Autodesk Fusion 360 part; units mm, degrees
(part 23 of 24)
  arc A327 (62.8291, 5.0441) -> (62.9009, 5.1159) centre (62.865, 5.08) ccw
  arc A328 (66.675, 5.0292) -> (66.675, 5.1308) centre (66.675, 5.08) ccw
  line L165 (33.655, 7.62) -> (32.385, 7.62)
  line L166 (34.29, 5.715) -> (34.925, 5.08)
  line L167 (36.195, 7.62) -> (34.925, 7.62)
  line L168 (64.135, 7.62) -> (62.865, 7.62)
  arc A329 (62.865, 7.6708) -> (62.865, 7.5692) centre (62.865, 7.62) ccw
  arc A330 (31.6992, 5.715) -> (31.8008, 5.715) centre (31.75, 5.715) ccw
  line L169 (56.515, 7.62) -> (55.245, 7.62)
  line L170 (57.785, 5.08) -> (59.055, 5.08)
  arc A331 (57.7491, 5.0441) -> (57.8209, 5.1159) centre (57.785, 5.08) ccw
  arc A332 (64.135, 7.5692) -> (64.135, 7.6708) centre (64.135, 7.62) ccw
  arc A333 (62.2659, 5.6791) -> (62.1941, 5.7509) centre (62.23, 5.715) ccw
  arc A334 (65.405, 7.6708) -> (65.405, 7.5692) centre (65.405, 7.62) ccw
  arc A335 (59.0909, 7.6559) -> (59.0191, 7.5841) centre (59.055, 7.62) ccw
  arc A336 (54.5741, 7.0209) -> (54.6459, 6.9491) centre (54.61, 6.985) ccw
  arc A337 (61.595, 7.5692) -> (61.595, 7.6708) centre (61.595, 7.62) ccw
  line L171 (60.325, 7.62) -> (59.69, 6.985)
  arc A338 (64.8059, 5.7509) -> (64.7341, 5.6791) centre (64.77, 5.715) ccw
  arc A339 (56.4791, 5.1159) -> (56.5509, 5.0441) centre (56.515, 5.08) ccw
  arc A340 (66.675, 7.5692) -> (66.675, 7.6708) centre (66.675, 7.62) ccw
  line L172 (62.865, 7.62) -> (62.23, 6.985)
  arc A341 (60.2891, 5.0441) -> (60.3609, 5.1159) centre (60.325, 5.08) ccw
  arc A342 (59.6541, 6.9491) -> (59.7259, 7.0209) centre (59.69, 6.985) ccw
  arc A343 (64.7341, 7.0209) -> (64.8059, 6.9491) centre (64.77, 6.985) ccw
  arc A344 (57.1141, 6.9491) -> (57.1859, 7.0209) centre (57.15, 6.985) ccw
  line L173 (60.325, 5.08) -> (61.595, 5.08)
  line L174 (59.69, 6.985) -> (59.055, 7.62)
  arc A345 (61.5591, 5.1159) -> (61.6309, 5.0441) centre (61.595, 5.08) ccw
  arc A346 (60.325, 5.1308) -> (60.325, 5.0292) centre (60.325, 5.08) ccw
  arc A347 (57.785, 5.1308) -> (57.785, 5.0292) centre (57.785, 5.08) ccw
  arc A348 (62.9009, 7.5841) -> (62.8291, 7.6559) centre (62.865, 7.62) ccw
  line L175 (66.675, 7.62) -> (65.405, 7.62)
  arc A349 (55.245, 7.6708) -> (55.245, 7.5692) centre (55.245, 7.62) ccw
  line L176 (61.595, 7.62) -> (60.325, 7.62)
  arc A350 (56.515, 7.5692) -> (56.515, 7.6708) centre (56.515, 7.62) ccw
  arc A351 (59.6541, 7.0209) -> (59.7259, 6.9491) centre (59.69, 6.985) ccw
  arc A352 (65.3691, 5.0441) -> (65.4409, 5.1159) centre (65.405, 5.08) ccw
  line L177 (61.595, 5.08) -> (62.23, 5.715)
  arc A353 (55.2091, 5.0441) -> (55.2809, 5.1159) centre (55.245, 5.08) ccw
  arc A354 (53.975, 5.0292) -> (53.975, 5.1308) centre (53.975, 5.08) ccw
  arc A355 (57.1141, 7.0209) -> (57.1859, 6.9491) centre (57.15, 6.985) ccw
  line L178 (64.77, 6.985) -> (65.405, 7.62)
  arc A356 (59.7259, 5.6791) -> (59.6541, 5.7509) centre (59.69, 5.715) ccw
  arc A357 (59.7259, 5.7509) -> (59.6541, 5.6791) centre (59.69, 5.715) ccw
  arc A358 (60.325, 7.6708) -> (60.325, 7.5692) centre (60.325, 7.62) ccw
  arc A359 (57.8209, 7.5841) -> (57.7491, 7.6559) centre (57.785, 7.62) ccw
  arc A360 (69.8141, 6.9491) -> (69.8859, 7.0209) centre (69.85, 6.985) ccw
  line L179 (62.23, 6.985) -> (61.595, 7.62)
  arc A361 (62.1941, 6.9491) -> (62.2659, 7.0209) centre (62.23, 6.985) ccw
  arc A362 (62.1941, 7.0209) -> (62.2659, 6.9491) centre (62.23, 6.985) ccw
  line L180 (57.15, 6.985) -> (57.785, 7.62)
  line L181 (57.785, 5.08) -> (57.15, 5.715)
  line L182 (55.245, 7.62) -> (54.61, 6.985)
  arc A363 (60.3609, 7.5841) -> (60.2891, 7.6559) centre (60.325, 7.62) ccw
  arc A364 (61.6309, 7.6559) -> (61.5591, 7.5841) centre (61.595, 7.62) ccw
  arc A365 (56.515, 5.0292) -> (56.515, 5.1308) centre (56.515, 5.08) ccw
  arc A366 (57.1859, 5.7509) -> (57.1141, 5.6791) centre (57.15, 5.715) ccw
  arc A367 (55.2809, 7.5841) -> (55.2091, 7.6559) centre (55.245, 7.62) ccw
  line L183 (65.405, 5.08) -> (64.77, 5.715)
sketch "Bottom Silkscreen" plane through (0, 0, 0) normal (0, 0, 1) x (1, 0, 0)
  arc A0 (64.6974, 49.0665) -> (64.6974, 49.1553) centre (64.6974, 49.1109) ccw
  arc A1 (63.764, 50.3111) -> (63.8529, 50.3111) centre (63.8085, 50.3111) ccw
  arc A2 (63.8084, 50.3111) -> (63.9418, 49.9999) centre (64.2381, 50.3111) ccw
  arc A3 (63.9756, 50.0287) -> (63.9079, 49.9711) centre (63.9418, 49.9999) ccw
  arc A4 (63.8529, 50.3111) -> (63.764, 50.311) centre (63.8085, 50.311) ccw
  arc A5 (65.4177, 49.4665) -> (65.7733, 49.1109) centre (65.7733, 49.4665) ccw
  arc A6 (64.6974, 50.3555) -> (64.2085, 50.7111) centre (64.2085, 50.1972) ccw
  arc A7 (65.4621, 49.4665) -> (65.3732, 49.4665) centre (65.4177, 49.4665) ccw
  arc A8 (65.7733, 49.1553) -> (65.7733, 49.0665) centre (65.7733, 49.1109) ccw
  line L0 (63.9418, 49.9999) -> (64.6974, 49.1109)
  arc A9 (64.2085, 50.7555) -> (64.2085, 50.6667) centre (64.2085, 50.7111) ccw
  arc A10 (64.6551, 50.3418) -> (64.7397, 50.3692) centre (64.6974, 50.3555) ccw
  arc A11 (64.6636, 49.0821) -> (64.7313, 49.1397) centre (64.6975, 49.1109) ccw
  line L1 (65.7733, 49.1109) -> (65.9511, 49.1109)
  arc A12 (63.8084, 49.1553) -> (63.8084, 49.0665) centre (63.8084, 49.1109) ccw
  arc A13 (65.9511, 49.0665) -> (65.9511, 49.1553) centre (65.9511, 49.1109) ccw
  arc A14 (63.9111, 49.9677) -> (63.9724, 50.0321) centre (63.9418, 49.9999) ccw
  arc A15 (64.2085, 50.7111) -> (63.8084, 50.3111) centre (64.2085, 50.311) ccw
  line L2 (64.6974, 49.1109) -> (63.8084, 49.1109)
  arc A16 (65.4621, 50.7111) -> (65.3732, 50.7111) centre (65.4177, 50.7111) ccw
  arc A17 (28.0289, 5.2134) -> (28.0289, 5.1244) centre (28.0289, 5.1689) ccw
  arc A18 (29.9938, 5.2134) -> (29.9938, 5.1244) centre (29.9938, 5.1689) ccw
  arc A19 (28.9179, 5.1244) -> (28.9179, 5.2134) centre (28.9179, 5.1689) ccw
  line L3 (29.9938, 5.1689) -> (30.1716, 5.1689)
  arc A20 (28.5179, 6.7691) -> (28.429, 6.7691) centre (28.4735, 6.7691) ccw
  arc A21 (29.6382, 5.5245) -> (29.9938, 5.1689) centre (29.9938, 5.5245) ccw
  arc A22 (28.5012, 6.8038) -> (28.4456, 6.7344) centre (28.4734, 6.7691) ccw
  line L4 (28.9179, 5.1689) -> (28.0289, 5.1689)
  line L5 (28.4734, 6.7691) -> (28.4734, 5.1689)
  arc A23 (29.9938, 5.1244) -> (29.9938, 5.2134) centre (29.9938, 5.1689) ccw
  arc A24 (28.429, 5.1689) -> (28.5179, 5.1689) centre (28.4735, 5.1689) ccw
  arc A25 (30.1716, 5.1244) -> (30.1716, 5.2134) centre (30.1716, 5.1689) ccw
  arc A26 (29.5937, 5.5245) -> (29.6826, 5.5245) centre (29.6382, 5.5245) ccw
  arc A27 (29.6826, 5.5245) -> (29.5937, 5.5245) centre (29.6382, 5.5245) ccw
  arc A28 (64.2085, 50.6667) -> (64.2085, 50.7555) centre (64.2085, 50.7111) ccw
  arc A29 (65.3732, 49.4665) -> (65.4621, 49.4665) centre (65.4177, 49.4665) ccw
  arc A30 (28.8901, 6.3788) -> (28.9457, 6.4482) centre (28.9179, 6.4135) ccw
  arc A31 (29.6826, 6.7691) -> (29.5937, 6.7691) centre (29.6382, 6.7691) ccw
  line L6 (65.4177, 50.7111) -> (65.4177, 49.4665)
  arc A32 (65.7733, 49.0665) -> (65.7733, 49.1553) centre (65.7733, 49.1109) ccw
  line L7 (29.6382, 6.7691) -> (29.6382, 5.5245)
  line L8 (28.9179, 6.4135) -> (28.4734, 6.7691)
sketch "Top Traces]" plane through (0, 0, 0) normal (0, 0, 1) x (1, 0, 0)
  arc A0 (58.4962, 25.4) -> (58.3438, 25.4) centre (58.42, 25.4) ccw
  arc A1 (31.6738, 22.86) -> (31.8262, 22.86) centre (31.75, 22.86) ccw
  line L0 (29.21, 10.16) -> (44.45, 10.16)
  arc A2 (26.67, 21.6662) -> (26.67, 21.5138) centre (26.67, 21.59) ccw
  arc A3 (30.48, 21.5138) -> (30.48, 21.6662) centre (30.48, 21.59) ccw
  line L1 (58.42, 16.51) -> (55.88, 13.97)
  arc A4 (29.21, 10.2362) -> (29.21, 10.0838) centre (29.21, 10.16) ccw
  arc A5 (44.5039, 10.2139) -> (44.3961, 10.1061) centre (44.45, 10.16) ccw
  line L2 (46.99, 11.43) -> (48.26, 10.16)
  arc A6 (45.6438, 6.35) -> (45.7962, 6.35) centre (45.72, 6.35) ccw
  arc A7 (58.4962, 20.32) -> (58.3438, 20.32) centre (58.42, 20.32) ccw
  arc A8 (46.99, 11.3538) -> (46.99, 11.5062) centre (46.99, 11.43) ccw
  line L3 (27.94, 16.51) -> (27.94, 19.05)
  arc A9 (25.3238, 13.97) -> (25.4762, 13.97) centre (25.4, 13.97) ccw
  arc A10 (48.3362, 10.16) -> (48.1838, 10.16) centre (48.26, 10.16) ccw
  arc A11 (28.0162, 19.05) -> (27.8638, 19.05) centre (27.94, 19.05) ccw
  line L4 (25.4, 13.97) -> (29.21, 10.16)
  line L5 (30.48, 11.43) -> (46.99, 11.43)
  line L6 (26.67, 21.59) -> (30.48, 21.59)
  arc A12 (25.3461, 20.3739) -> (25.4539, 20.2661) centre (25.4, 20.32) ccw
  line L7 (55.88, 13.97) -> (45.72, 13.97)
  arc A13 (48.2061, 10.1061) -> (48.3139, 10.2139) centre (48.26, 10.16) ccw
  arc A14 (25.3238, 16.51) -> (25.4762, 16.51) centre (25.4, 16.51) ccw
  arc A15 (58.3438, 16.51) -> (58.4962, 16.51) centre (58.42, 16.51) ccw
  line L8 (58.42, 20.32) -> (58.42, 16.51)
  arc A16 (26.7239, 21.5361) -> (26.6161, 21.6439) centre (26.67, 21.59) ccw
  line L9 (27.94, 13.97) -> (30.48, 11.43)
  arc A17 (44.45, 10.0838) -> (44.45, 10.2362) centre (44.45, 10.16) ccw
  arc A18 (45.7962, 8.89) -> (45.6438, 8.89) centre (45.72, 8.89) ccw
  arc A19 (30.4261, 21.6439) -> (30.5339, 21.5361) centre (30.48, 21.59) ccw
  arc A20 (25.4539, 14.0239) -> (25.3461, 13.9161) centre (25.4, 13.97) ccw
  line L10 (27.94, 16.51) -> (27.94, 13.97)
  arc A21 (29.1561, 10.1061) -> (29.2639, 10.2139) centre (29.21, 10.16) ccw
  arc A22 (31.8039, 22.8061) -> (31.6961, 22.9139) centre (31.75, 22.86) ccw
  line L11 (44.45, 10.16) -> (45.72, 8.89)
  arc A23 (63.6587, 35.56) -> (63.3413, 35.56) centre (63.5, 35.56) ccw
  line L12 (25.4, 16.51) -> (25.4, 13.97)
  arc A24 (55.88, 13.8938) -> (55.88, 14.0462) centre (55.88, 13.97) ccw
  line L13 (25.4, 16.51) -> (25.4, 20.32)
  line L14 (30.48, 21.59) -> (31.75, 22.86)
  arc A25 (27.9939, 14.0239) -> (27.8861, 13.9161) centre (27.94, 13.97) ccw
  arc A26 (30.4261, 11.3761) -> (30.5339, 11.4839) centre (30.48, 11.43) ccw
  arc A27 (45.72, 14.0462) -> (45.72, 13.8938) centre (45.72, 13.97) ccw
  line L15 (45.72, 8.89) -> (45.72, 6.35)
  line L16 (31.75, 22.86) -> (31.75, 25.4)
  arc A28 (25.4762, 16.51) -> (25.3238, 16.51) centre (25.4, 16.51) ccw
  line L17 (25.4, 20.32) -> (26.67, 21.59)
  arc A29 (27.8638, 16.51) -> (28.0162, 16.51) centre (27.94, 16.51) ccw
  arc A30 (47.0439, 11.4839) -> (46.9361, 11.3761) centre (46.99, 11.43) ccw
  arc A31 (58.4739, 16.4561) -> (58.3661, 16.5639) centre (58.42, 16.51) ccw
  arc A32 (15.8897, 25.7957) -> (16.1143, 26.0203) centre (16.002, 25.908) ccw
  arc A33 (30.48, 11.5062) -> (30.48, 11.3538) centre (30.48, 11.43) ccw
  arc A34 (40.7987, 38.1) -> (40.4813, 38.1) centre (40.64, 38.1) ccw
  arc A35 (48.1838, 6.35) -> (48.3362, 6.35) centre (48.26, 6.35) ccw
  arc A36 (15.3523, 26.7823) -> (15.1277, 26.5577) centre (15.24, 26.67) ccw
  arc A37 (45.6661, 8.8361) -> (45.7739, 8.9439) centre (45.72, 8.89) ccw
  arc A38 (28.0162, 16.51) -> (27.8638, 16.51) centre (27.94, 16.51) ccw
  line L18 (58.42, 25.4) -> (58.42, 20.32)
  line L19 (48.26, 10.16) -> (48.26, 6.35)
  arc A39 (30.5562, 17.78) -> (30.4038, 17.78) centre (30.48, 17.78) ccw
  line L20 (49.53, 12.7) -> (50.8, 11.43)
  arc A40 (31.8231, 20.3739) -> (31.9309, 20.2661) centre (31.877, 20.32) ccw
  line L21 (31.75, 12.7) -> (49.53, 12.7)
  line L22 (76.2, 29.718) -> (75.692, 29.21)
  arc A41 (70.0309, 29.1561) -> (69.9231, 29.2639) centre (69.977, 29.21) ccw
  arc A42 (36.9062, 25.4) -> (36.7538, 25.4) centre (36.83, 25.4) ccw
  line L23 (30.48, 16.51) -> (30.48, 13.97)
  arc A43 (33.02, 18.9738) -> (33.02, 19.1262) centre (33.02, 19.05) ccw
  arc A44 (55.8261, 14.0239) -> (55.9339, 13.9161) centre (55.88, 13.97) ccw
  arc A45 (36.8839, 22.8061) -> (36.7761, 22.9139) centre (36.83, 22.86) ccw
  line L24 (31.75, 19.05) -> (33.02, 19.05)
  line L25 (60.96, 25.4) -> (60.96, 15.24)
  arc A46 (30.5562, 16.51) -> (30.4038, 16.51) centre (30.48, 16.51) ccw
  arc A47 (25.4762, 20.32) -> (25.3238, 20.32) centre (25.4, 20.32) ccw
  arc A48 (61.0362, 25.4) -> (60.8838, 25.4) centre (60.96, 25.4) ccw
  arc A49 (30.4261, 17.8339) -> (30.5339, 17.7261) centre (30.48, 17.78) ccw
  line L26 (33.02, 19.05) -> (36.83, 22.86)
  arc A50 (50.8762, 11.43) -> (50.7238, 11.43) centre (50.8, 11.43) ccw
  line L27 (34.29, 22.733) -> (34.29, 25.4)
  arc A51 (50.7238, 6.35) -> (50.8762, 6.35) centre (50.8, 6.35) ccw
  line L28 (76.2, 31.75) -> (76.2, 29.718)
  arc A52 (34.3439, 22.6791) -> (34.2361, 22.7869) centre (34.29, 22.733) ccw
  arc A53 (27.8861, 19.1039) -> (27.9939, 18.9961) centre (27.94, 19.05) ccw
  line L29 (75.692, 29.21) -> (69.977, 29.21)
  arc A54 (58.3438, 20.32) -> (58.4962, 20.32) centre (58.42, 20.32) ccw
  arc A55 (31.8262, 25.4) -> (31.6738, 25.4) centre (31.75, 25.4) ccw
  arc A56 (75.6381, 29.2639) -> (75.7459, 29.1561) centre (75.692, 29.21) ccw
  arc A57 (76.2762, 31.75) -> (76.1238, 31.75) centre (76.2, 31.75) ccw
  line L30 (31.877, 20.32) -> (34.29, 22.733)
  line L31 (30.48, 13.97) -> (31.75, 12.7)
  arc A58 (58.3661, 12.7539) -> (58.4739, 12.6461) centre (58.42, 12.7) ccw
  arc A59 (61.0139, 15.1861) -> (60.9061, 15.2939) centre (60.96, 15.24) ccw
  arc A60 (69.2881, 28.6289) -> (69.3959, 28.5211) centre (69.342, 28.575) ccw
  arc A61 (30.4038, 13.97) -> (30.5562, 13.97) centre (30.48, 13.97) ccw
  arc A62 (27.8638, 13.97) -> (28.0162, 13.97) centre (27.94, 13.97) ccw
  arc A63 (29.2639, 20.2661) -> (29.1561, 20.3739) centre (29.21, 20.32) ccw
  line L32 (58.42, 12.7) -> (55.88, 12.7)
  arc A64 (49.53, 12.6238) -> (49.53, 12.7762) centre (49.53, 12.7) ccw
  arc A65 (49.5839, 12.7539) -> (49.4761, 12.6461) centre (49.53, 12.7) ccw
  arc A66 (75.692, 29.1338) -> (75.692, 29.2862) centre (75.692, 29.21) ccw
  arc A67 (69.977, 29.2862) -> (69.977, 29.1338) centre (69.977, 29.21) ccw
  arc A68 (31.75, 19.1262) -> (31.75, 18.9738) centre (31.75, 19.05) ccw
  line L33 (69.977, 29.21) -> (69.342, 28.575)
  line L34 (60.96, 15.24) -> (58.42, 12.7)
  line L35 (30.48, 17.78) -> (31.75, 19.05)
  arc A69 (50.7461, 11.3761) -> (50.8539, 11.4839) centre (50.8, 11.43) ccw
  line L36 (30.48, 16.51) -> (30.48, 17.78)
  line L37 (36.83, 22.86) -> (36.83, 25.4)
  arc A70 (31.877, 20.2438) -> (31.877, 20.3962) centre (31.877, 20.32) ccw
  arc A71 (31.8039, 18.9961) -> (31.6961, 19.1039) centre (31.75, 19.05) ccw
  arc A72 (76.1238, 29.718) -> (76.2762, 29.718) centre (76.2, 29.718) ccw
  arc A73 (34.3662, 25.4) -> (34.2138, 25.4) centre (34.29, 25.4) ccw
  arc A74 (36.7538, 22.86) -> (36.9062, 22.86) centre (36.83, 22.86) ccw
  arc A75 (32.9661, 19.1039) -> (33.0739, 18.9961) centre (33.02, 19.05) ccw
  arc A76 (60.8838, 15.24) -> (61.0362, 15.24) centre (60.96, 15.24) ccw
  arc A77 (34.2138, 22.733) -> (34.3662, 22.733) centre (34.29, 22.733) ccw
  arc A78 (76.2539, 29.6641) -> (76.1461, 29.7719) centre (76.2, 29.718) ccw
  arc A79 (29.21, 20.3962) -> (29.21, 20.2438) centre (29.21, 20.32) ccw
  line L38 (27.94, 19.05) -> (29.21, 20.32)
  arc A80 (62.1761, 24.1839) -> (62.2839, 24.0761) centre (62.23, 24.13) ccw
  line L39 (76.2, 40.64) -> (76.2, 44.45)
  arc A81 (76.2539, 40.5861) -> (76.1461, 40.6939) centre (76.2, 40.64) ccw
  arc A82 (60.9061, 25.4539) -> (61.0139, 25.3461) centre (60.96, 25.4) ccw
  line L40 (55.88, 10.16) -> (57.15, 11.43)
  line L41 (62.23, 13.97) -> (62.23, 24.13)
  arc A83 (62.1538, 13.97) -> (62.3062, 13.97) centre (62.23, 13.97) ccw
  line L42 (50.8, 11.43) -> (50.8, 6.35)
  line L43 (65.405, 27.305) -> (70.485, 27.305)
  line L44 (69.342, 28.575) -> (64.135, 28.575)
  line L45 (57.15, 11.43) -> (59.69, 11.43)
  arc A84 (76.2762, 44.45) -> (76.1238, 44.45) centre (76.2, 44.45) ccw
  arc A85 (77.4161, 27.9939) -> (77.5239, 27.8861) centre (77.47, 27.94) ccw
  arc A86 (58.42, 12.6238) -> (58.42, 12.7762) centre (58.42, 12.7) ccw
  line L46 (53.34, 10.16) -> (53.34, 6.35)
  arc A87 (74.8761, 39.4239) -> (74.9839, 39.3161) centre (74.93, 39.37) ccw
  line L47 (71.12, 39.37) -> (74.93, 39.37)
  line L48 (55.88, 6.35) -> (55.88, 10.16)
  arc A88 (57.15, 11.5062) -> (57.15, 11.3538) centre (57.15, 11.43) ccw
  arc A89 (62.2839, 13.9161) -> (62.1761, 14.0239) centre (62.23, 13.97) ccw
  arc A90 (74.93, 39.2938) -> (74.93, 39.4462) centre (74.93, 39.37) ccw
  arc A91 (55.9562, 10.16) -> (55.8038, 10.16) centre (55.88, 10.16) ccw
  line L49 (29.21, 20.32) -> (31.877, 20.32)
  arc A92 (64.1889, 28.5211) -> (64.0811, 28.6289) centre (64.135, 28.575) ccw
  arc A93 (53.2861, 10.2139) -> (53.3939, 10.1061) centre (53.34, 10.16) ccw
  arc A94 (71.12, 39.4462) -> (71.12, 39.2938) centre (71.12, 39.37) ccw
  arc A95 (76.1238, 40.64) -> (76.2762, 40.64) centre (76.2, 40.64) ccw
  arc A96 (65.4589, 27.2511) -> (65.3511, 27.3589) centre (65.405, 27.305) ccw
  line L50 (62.23, 24.13) -> (65.405, 27.305)
  arc A97 (71.1739, 27.8861) -> (71.0661, 27.9939) centre (71.12, 27.94) ccw
  arc A98 (30.4038, 16.51) -> (30.5562, 16.51) centre (30.48, 16.51) ccw
  line L51 (70.485, 27.305) -> (71.12, 27.94)
  arc A99 (70.485, 27.2288) -> (70.485, 27.3812) centre (70.485, 27.305) ccw
  arc A100 (77.47, 27.8638) -> (77.47, 28.0162) centre (77.47, 27.94) ccw
  line L52 (55.88, 12.7) -> (53.34, 10.16)
  arc A101 (59.69, 11.3538) -> (59.69, 11.5062) centre (59.69, 11.43) ccw
  arc A102 (59.6361, 11.4839) -> (59.7439, 11.3761) centre (59.69, 11.43) ccw
  arc A103 (55.88, 12.7762) -> (55.88, 12.6238) centre (55.88, 12.7) ccw
  arc A104 (64.135, 28.6512) -> (64.135, 28.4988) centre (64.135, 28.575) ccw
  arc A105 (55.8038, 6.35) -> (55.9562, 6.35) centre (55.88, 6.35) ccw
  arc A106 (31.75, 12.7762) -> (31.75, 12.6238) centre (31.75, 12.7) ccw
  arc A107 (69.342, 28.4988) -> (69.342, 28.6512) centre (69.342, 28.575) ccw
  arc A108 (55.8261, 10.2139) -> (55.9339, 10.1061) centre (55.88, 10.16) ccw
  arc A109 (30.5339, 14.0239) -> (30.4261, 13.9161) centre (30.48, 13.97) ccw
  arc A110 (62.3062, 24.13) -> (62.1538, 24.13) centre (62.23, 24.13) ccw
  arc A111 (31.6961, 12.6461) -> (31.8039, 12.7539) centre (31.75, 12.7) ccw
  arc A112 (53.4162, 10.16) -> (53.2638, 10.16) centre (53.34, 10.16) ccw
  arc A113 (55.9339, 12.6461) -> (55.8261, 12.7539) centre (55.88, 12.7) ccw
  arc A114 (65.405, 27.3812) -> (65.405, 27.2288) centre (65.405, 27.305) ccw
  arc A115 (53.2638, 6.35) -> (53.4162, 6.35) centre (53.34, 6.35) ccw
  arc A116 (70.4311, 27.3589) -> (70.5389, 27.2511) centre (70.485, 27.305) ccw
  line L53 (64.135, 28.575) -> (60.96, 25.4)
  line L54 (74.93, 39.37) -> (76.2, 40.64)
  arc A117 (57.2039, 11.3761) -> (57.0961, 11.4839) centre (57.15, 11.43) ccw
  line L55 (59.69, 11.43) -> (62.23, 13.97)
  line L56 (71.12, 27.94) -> (77.47, 27.94)
  line L57 (3.048, 46.228) -> (3.81, 46.99)
  line L58 (3.81, 46.99) -> (8.89, 46.99)
  arc A118 (60.96, 31.6738) -> (60.96, 31.8262) centre (60.96, 31.75) ccw
  arc A119 (55.8038, 34.29) -> (55.9562, 34.29) centre (55.88, 34.29) ccw
  line L59 (60.96, 31.75) -> (54.61, 31.75)
  line L60 (3.048, 44.45) -> (3.048, 46.228)
  arc A120 (16.5862, 49.53) -> (16.4338, 49.53) centre (16.51, 49.53) ccw
  line L61 (76.327, 36.83) -> (78.74, 39.243)
  arc A121 (10.16, 45.7962) -> (10.16, 45.6438) centre (10.16, 45.72) ccw
  line L62 (15.24, 45.72) -> (16.51, 46.99)
  arc A122 (71.12, 36.9062) -> (71.12, 36.7538) centre (71.12, 36.83) ccw
  arc A123 (76.327, 36.7538) -> (76.327, 36.9062) centre (76.327, 36.83) ccw
  arc A124 (78.6638, 39.243) -> (78.8162, 39.243) centre (78.74, 39.243) ccw
  line L63 (71.12, 36.83) -> (76.327, 36.83)
  line L64 (67.31, 16.51) -> (67.31, 10.16)
  arc A125 (78.8162, 44.45) -> (78.6638, 44.45) centre (78.74, 44.45) ccw
  arc A126 (78.6638, 29.21) -> (78.8162, 29.21) centre (78.74, 29.21) ccw
  arc A127 (8.89, 46.9138) -> (8.89, 47.0662) centre (8.89, 46.99) ccw
  arc A128 (3.1242, 46.228) -> (2.9718, 46.228) centre (3.048, 46.228) ccw
  arc A129 (2.9718, 44.45) -> (3.1242, 44.45) centre (3.048, 44.45) ccw
  line L65 (77.47, 27.94) -> (78.74, 29.21)
  arc A130 (3.81, 47.0662) -> (3.81, 46.9138) centre (3.81, 46.99) ccw
  line L66 (8.89, 46.99) -> (10.16, 45.72)
  arc A131 (15.24, 45.6438) -> (15.24, 45.7962) centre (15.24, 45.72) ccw
  arc A132 (76.2731, 36.8839) -> (76.3809, 36.7761) centre (76.327, 36.83) ccw
  arc A133 (67.3862, 16.51) -> (67.2338, 16.51) centre (67.31, 16.51) ccw
  arc A134 (53.3939, 33.0739) -> (53.2861, 32.9661) centre (53.34, 33.02) ccw
  arc A135 (53.4162, 49.53) -> (53.2638, 49.53) centre (53.34, 49.53) ccw
  line L67 (53.34, 44.45) -> (53.34, 33.02)
  arc A136 (54.61, 31.8262) -> (54.61, 31.6738) centre (54.61, 31.75) ccw
  line L68 (78.74, 29.21) -> (78.74, 31.75)
  arc A137 (3.8639, 46.9361) -> (3.7561, 47.0439) centre (3.81, 46.99) ccw
  arc A138 (78.7939, 29.1561) -> (78.6861, 29.2639) centre (78.74, 29.21) ccw
  line L69 (54.61, 31.75) -> (53.34, 33.02)
  arc A139 (53.2638, 44.45) -> (53.4162, 44.45) centre (53.34, 44.45) ccw
  arc A140 (16.5639, 46.9361) -> (16.4561, 47.0439) centre (16.51, 46.99) ccw
  arc A141 (35.5061, 16.5639) -> (35.6139, 16.4561) centre (35.56, 16.51) ccw
  arc A142 (78.8162, 31.75) -> (78.6638, 31.75) centre (78.74, 31.75) ccw
  arc A143 (78.7939, 39.1891) -> (78.6861, 39.2969) centre (78.74, 39.243) ccw
  arc A144 (53.4162, 44.45) -> (53.2638, 44.45) centre (53.34, 44.45) ccw
  line L70 (38.735, 32.385) -> (40.64, 30.48)
  arc A145 (38.8112, 43.18) -> (38.6588, 43.18) centre (38.735, 43.18) ccw
  arc A146 (63.4238, 43.18) -> (63.5762, 43.18) centre (63.5, 43.18) ccw
  arc A147 (15.1861, 45.7739) -> (15.2939, 45.6661) centre (15.24, 45.72) ccw
  arc A148 (55.9562, 49.53) -> (55.8038, 49.53) centre (55.88, 49.53) ccw
  line L71 (78.74, 39.243) -> (78.74, 44.45)
  arc A149 (53.2638, 33.02) -> (53.4162, 33.02) centre (53.34, 33.02) ccw
  arc A150 (54.5561, 31.6961) -> (54.6639, 31.8039) centre (54.61, 31.75) ccw
  arc A151 (8.9439, 47.0439) -> (8.8361, 46.9361) centre (8.89, 46.99) ccw
  line L72 (10.16, 45.72) -> (15.24, 45.72)
  line L73 (53.34, 49.53) -> (53.34, 44.45)
  arc A152 (2.9941, 46.2819) -> (3.1019, 46.1741) centre (3.048, 46.228) ccw
  arc A153 (71.12, 28.0162) -> (71.12, 27.8638) centre (71.12, 27.94) ccw
  arc A154 (10.1061, 45.6661) -> (10.2139, 45.7739) centre (10.16, 45.72) ccw
  arc A155 (16.4338, 46.99) -> (16.5862, 46.99) centre (16.51, 46.99) ccw
  arc A156 (67.2338, 10.16) -> (67.3862, 10.16) centre (67.31, 10.16) ccw
  line L74 (16.51, 46.99) -> (16.51, 49.53)
  line L75 (55.88, 49.53) -> (55.88, 34.29)
  arc A157 (34.3439, 33.0739) -> (34.2361, 32.9661) centre (34.29, 33.02) ccw
  arc A158 (34.3662, 34.29) -> (34.2138, 34.29) centre (34.29, 34.29) ccw
  arc A159 (44.5262, 43.18) -> (44.3738, 43.18) centre (44.45, 43.18) ccw
  arc A160 (32.9661, 16.5639) -> (33.0739, 16.4561) centre (33.02, 16.51) ccw
  arc A161 (34.2138, 33.02) -> (34.3662, 33.02) centre (34.29, 33.02) ccw
  line L76 (35.56, 16.51) -> (44.45, 25.4)
  arc A162 (39.2938, 22.86) -> (39.4462, 22.86) centre (39.37, 22.86) ccw
  arc A163 (63.4461, 53.2861) -> (63.5539, 53.3939) centre (63.5, 53.34) ccw
  arc A164 (40.7162, 52.07) -> (40.5638, 52.07) centre (40.64, 52.07) ccw
  line L77 (62.23, 54.61) -> (63.5, 53.34)
  arc A165 (38.0238, 43.815) -> (38.1762, 43.815) centre (38.1, 43.815) ccw
  arc A166 (44.3961, 43.1261) -> (44.5039, 43.2339) centre (44.45, 43.18) ccw
  arc A167 (62.2839, 54.6639) -> (62.1761, 54.5561) centre (62.23, 54.61) ccw
  line L78 (34.29, 33.02) -> (34.29, 34.29)
  line L79 (44.45, 43.18) -> (40.64, 46.99)
  arc A168 (38.7889, 32.4389) -> (38.6811, 32.3311) centre (38.735, 32.385) ccw
  arc A169 (44.3738, 25.4) -> (44.5262, 25.4) centre (44.45, 25.4) ccw
  arc A170 (40.6939, 47.0439) -> (40.5861, 46.9361) centre (40.64, 46.99) ccw
  line L80 (40.64, 49.53) -> (40.64, 52.07)
  arc A171 (38.1762, 49.53) -> (38.0238, 49.53) centre (38.1, 49.53) ccw
  line L81 (38.735, 43.18) -> (38.735, 32.385)
  arc A172 (43.2339, 54.5561) -> (43.1261, 54.6639) centre (43.18, 54.61) ccw
  line L82 (40.64, 46.99) -> (40.64, 49.53)
  arc A173 (40.7162, 49.53) -> (40.5638, 49.53) centre (40.64, 49.53) ccw
  line L83 (43.18, 54.61) -> (62.23, 54.61)
  arc A174 (38.1539, 43.8689) -> (38.0461, 43.7611) centre (38.1, 43.815) ccw
  line L84 (38.1, 49.53) -> (38.1, 43.815)
  arc A175 (39.4239, 22.8061) -> (39.3161, 22.9139) centre (39.37, 22.86) ccw
  arc A176 (38.6588, 32.385) -> (38.8112, 32.385) centre (38.735, 32.385) ccw
  arc A177 (38.6811, 43.1261) -> (38.7889, 43.2339) centre (38.735, 43.18) ccw
  arc A178 (40.5638, 49.53) -> (40.7162, 49.53) centre (40.64, 49.53) ccw
  arc A179 (63.5762, 53.34) -> (63.4238, 53.34) centre (63.5, 53.34) ccw
  arc A180 (40.5861, 30.4261) -> (40.6939, 30.5339) centre (40.64, 30.48) ccw
  arc A181 (62.23, 54.5338) -> (62.23, 54.6862) centre (62.23, 54.61) ccw
  line L85 (63.5, 43.18) -> (63.5, 53.34)
  arc A182 (43.18, 54.6862) -> (43.18, 54.5338) centre (43.18, 54.61) ccw
  line L86 (39.37, 27.94) -> (34.29, 33.02)
  arc A183 (40.5638, 46.99) -> (40.7162, 46.99) centre (40.64, 46.99) ccw
  line L87 (33.02, 16.51) -> (39.37, 22.86)
  line L88 (44.45, 25.4) -> (44.45, 43.18)
  line L89 (39.37, 22.86) -> (39.37, 27.94)
  arc A184 (39.3161, 27.8861) -> (39.4239, 27.9939) centre (39.37, 27.94) ccw
  arc A185 (44.5039, 25.3461) -> (44.3961, 25.4539) centre (44.45, 25.4) ccw
  line L90 (40.64, 52.07) -> (43.18, 54.61)
  arc A186 (39.4462, 27.94) -> (39.2938, 27.94) centre (39.37, 27.94) ccw
  line L91 (38.1, 43.815) -> (38.735, 43.18)
  arc A187 (40.5861, 52.1239) -> (40.6939, 52.0161) centre (40.64, 52.07) ccw
  arc A188 (24.6888, 29.21) -> (24.8412, 29.21) centre (24.765, 29.21) ccw
  arc A189 (32.9438, 43.18) -> (33.0962, 43.18) centre (33.02, 43.18) ccw
  arc A190 (15.24, 21.4312) -> (15.24, 21.7488) centre (15.24, 21.59) ccw
  line L92 (72.009, 23.749) -> (72.009, 14.224)
  arc A191 (33.0739, 43.2339) -> (32.9661, 43.1261) centre (33.02, 43.18) ccw
  arc A192 (34.2361, 41.8561) -> (34.3439, 41.9639) centre (34.29, 41.91) ccw
  arc A193 (24.8412, 45.72) -> (24.6888, 45.72) centre (24.765, 45.72) ccw
  line L93 (34.29, 41.91) -> (36.83, 41.91)
  arc A194 (33.0962, 49.53) -> (32.9438, 49.53) centre (33.02, 49.53) ccw
  arc A195 (7.62, 21.7488) -> (7.62, 21.4312) centre (7.62, 21.59) ccw
  line L94 (33.02, 43.18) -> (34.29, 41.91)
  arc A196 (72.3583, 12.446) -> (72.6758, 12.446) centre (72.517, 12.446) ccw
  line L95 (20.32, 35.56) -> (17.78, 33.02)
  line L96 (66.04, 31.75) -> (66.04, 43.18)
  line L97 (72.517, 13.716) -> (72.517, 12.446)
  arc A197 (17.9388, 33.02) -> (17.6212, 33.02) centre (17.78, 33.02) ccw
  line L98 (17.78, 33.02) -> (17.78, 24.13)
  arc A198 (72.2313, 24.13) -> (72.5487, 24.13) centre (72.39, 24.13) ccw
  line L99 (20.32, 38.1) -> (20.32, 35.56)
  line L100 (19.431, 44.069) -> (13.97, 44.069)
  arc A199 (17.6677, 33.1323) -> (17.8923, 32.9077) centre (17.78, 33.02) ccw
  arc A200 (71.8503, 14.224) -> (72.1677, 14.224) centre (72.009, 14.224) ccw
  line L101 (17.78, 24.13) -> (15.24, 21.59)
  arc A201 (72.1213, 14.3363) -> (71.8967, 14.1117) centre (72.009, 14.224) ccw
  arc A202 (72.5023, 24.0177) -> (72.2777, 24.2423) centre (72.39, 24.13) ccw
  arc A203 (53.1813, 17.78) -> (53.4988, 17.78) centre (53.3401, 17.78) ccw
  arc A204 (72.4047, 13.6037) -> (72.6293, 13.8283) centre (72.517, 13.716) ccw
  arc A205 (72.6758, 13.716) -> (72.3583, 13.716) centre (72.517, 13.716) ccw
  arc A206 (17.8923, 24.0177) -> (17.6677, 24.2423) centre (17.78, 24.13) ccw
  arc A207 (66.1988, 43.18) -> (65.8813, 43.18) centre (66.0401, 43.18) ccw
  line L102 (15.24, 21.59) -> (7.62, 21.59)
  arc A208 (13.97, 44.1452) -> (13.97, 43.9928) centre (13.97, 44.069) ccw
  arc A209 (15.1277, 21.7023) -> (15.3523, 21.4777) centre (15.24, 21.59) ccw
  line L103 (72.517, 13.716) -> (72.009, 14.224)
  arc A210 (19.431, 43.9928) -> (19.431, 44.1452) centre (19.431, 44.069) ccw
  line L104 (33.02, 49.53) -> (33.02, 43.18)
  arc A211 (36.83, 41.8338) -> (36.83, 41.9862) centre (36.83, 41.91) ccw
  line L105 (24.765, 45.72) -> (24.765, 29.21)
  arc A212 (34.29, 41.9862) -> (34.29, 41.8338) centre (34.29, 41.91) ccw
  line L106 (23.241, 44.069) -> (21.59, 45.72)
  arc A213 (19.4849, 44.1229) -> (19.3771, 44.0151) centre (19.431, 44.069) ccw
  arc A214 (65.8813, 31.75) -> (66.1988, 31.75) centre (66.0401, 31.75) ccw
  arc A215 (20.1612, 35.56) -> (20.4788, 35.56) centre (20.32, 35.56) ccw
  line L107 (72.39, 24.13) -> (72.009, 23.749)
  arc A216 (72.5487, 25.4) -> (72.2313, 25.4) centre (72.39, 25.4) ccw
  arc A217 (20.4788, 38.1) -> (20.1612, 38.1) centre (20.32, 38.1) ccw
  arc A218 (53.4988, 25.4) -> (53.1813, 25.4) centre (53.3401, 25.4) ccw
  arc A219 (20.4323, 35.4477) -> (20.2077, 35.6723) centre (20.32, 35.56) ccw
  line L108 (28.575, 36.195) -> (35.4838, 36.195)
  arc A220 (28.6289, 36.1411) -> (28.5211, 36.2489) centre (28.575, 36.195) ccw
  line L109 (20.32, 33.02) -> (20.32, 20.32)
  arc A221 (41.8338, 25.4) -> (41.9862, 25.4) centre (41.91, 25.4) ccw
  arc A222 (26.6161, 34.3439) -> (26.7239, 34.2361) centre (26.67, 34.29) ccw
  arc A223 (36.7538, 32.258) -> (36.9062, 32.258) centre (36.83, 32.258) ccw
  line L110 (35.4838, 36.195) -> (36.83, 34.8488)
  arc A224 (20.2077, 33.1323) -> (20.4323, 32.9077) centre (20.32, 33.02) ccw
  arc A225 (36.8839, 32.3119) -> (36.7761, 32.2041) centre (36.83, 32.258) ccw
  arc A226 (23.1287, 43.9567) -> (23.3533, 44.1813) centre (23.241, 44.069) ccw
  arc A227 (20.1612, 20.32) -> (20.4788, 20.32) centre (20.32, 20.32) ccw
  arc A228 (36.7761, 34.7949) -> (36.8839, 34.9027) centre (36.83, 34.8488) ccw
  arc A229 (35.5377, 36.2489) -> (35.4299, 36.1411) centre (35.4838, 36.195) ccw
  arc A230 (20.4323, 20.2077) -> (20.2077, 20.4323) centre (20.32, 20.32) ccw
  line L111 (23.241, 35.941) -> (20.32, 33.02)
  arc A231 (28.575, 36.2712) -> (28.575, 36.1188) centre (28.575, 36.195) ccw
  line L112 (26.67, 34.29) -> (28.575, 36.195)
  arc A232 (36.9062, 34.8488) -> (36.7538, 34.8488) centre (36.83, 34.8488) ccw
  line L113 (21.59, 49.53) -> (21.59, 45.72)
  arc A233 (20.2661, 43.1261) -> (20.3739, 43.2339) centre (20.32, 43.18) ccw
  arc A234 (15.1277, 15.3523) -> (15.3523, 15.1277) centre (15.24, 15.24) ccw
  arc A235 (23.3533, 35.8287) -> (23.1287, 36.0533) centre (23.241, 35.941) ccw
  arc A236 (35.4838, 36.1188) -> (35.4838, 36.2712) centre (35.4838, 36.195) ccw
  arc A237 (21.7023, 45.8323) -> (21.4777, 45.6077) centre (21.59, 45.72) ccw
  arc A238 (71.8967, 23.8613) -> (72.1213, 23.6367) centre (72.009, 23.749) ccw
  arc A239 (23.3998, 44.069) -> (23.0822, 44.069) centre (23.241, 44.069) ccw
  arc A240 (72.1677, 23.749) -> (71.8503, 23.749) centre (72.009, 23.749) ccw
  arc A241 (41.9862, 27.178) -> (41.8338, 27.178) centre (41.91, 27.178) ccw
  line L114 (36.83, 34.8488) -> (36.83, 32.258)
  line L115 (41.91, 27.178) -> (41.91, 25.4)
  arc A242 (21.4312, 45.72) -> (21.7488, 45.72) centre (21.59, 45.72) ccw
  line L116 (20.32, 20.32) -> (15.24, 15.24)
  arc A243 (20.4788, 33.02) -> (20.1612, 33.02) centre (20.32, 33.02) ccw
  line L117 (53.34, 25.4) -> (53.34, 17.78)
  line L118 (23.241, 44.069) -> (23.241, 35.941)
  line L119 (72.39, 25.4) -> (72.39, 24.13)
  line L120 (41.91, 27.178) -> (36.83, 32.258)
  line L121 (19.431, 44.069) -> (20.32, 43.18)
  arc A244 (41.8561, 27.1241) -> (41.9639, 27.2319) centre (41.91, 27.178) ccw
  arc A245 (17.6212, 24.13) -> (17.9388, 24.13) centre (17.78, 24.13) ccw
  arc A246 (23.0822, 35.941) -> (23.3998, 35.941) centre (23.241, 35.941) ccw
  arc A247 (21.7488, 49.53) -> (21.4312, 49.53) centre (21.59, 49.53) ccw
  arc A248 (72.5487, 8.89) -> (72.2313, 8.89) centre (72.39, 8.89) ccw
  arc A249 (72.5023, 3.9223) -> (72.2777, 3.6977) centre (72.39, 3.81) ccw
  arc A250 (63.3877, 35.4477) -> (63.6123, 35.6723) centre (63.5, 35.56) ccw
  line L122 (22.86, 16.51) -> (22.86, 24.13)
  arc A251 (63.3413, 31.75) -> (63.6587, 31.75) centre (63.5, 31.75) ccw
  line L123 (73.66, 10.16) -> (74.93, 10.16)
  arc A252 (73.3171, 3.0417) -> (73.3171, 2.7242) centre (73.3171, 2.883) ccw
  arc A253 (72.2313, 3.81) -> (72.5487, 3.81) centre (72.39, 3.81) ccw
  arc A254 (74.93, 10.0013) -> (74.93, 10.3187) centre (74.93, 10.16) ccw
  arc A255 (74.8177, 10.2723) -> (75.0423, 10.0477) centre (74.93, 10.16) ccw
  arc A256 (72.2777, 9.0023) -> (72.5023, 8.7777) centre (72.39, 8.89) ccw
  arc A257 (74.2467, 2.7242) -> (74.2467, 3.0417) centre (74.2467, 2.883) ccw
  arc A258 (76.0413, 11.43) -> (76.3588, 11.43) centre (76.2001, 11.43) ccw
  line L124 (72.39, 8.89) -> (73.66, 10.16)
  line L125 (76.2, 14.8082) -> (74.2188, 16.7894)
  line L126 (72.39, 3.81) -> (72.39, 8.89)
  line L127 (76.2, 11.43) -> (76.2, 14.8082)
  line L128 (50.8, 25.4) -> (50.8, 17.78)
  arc A259 (50.9588, 25.4) -> (50.6413, 25.4) centre (50.8001, 25.4) ccw
  arc A260 (73.2048, 2.7706) -> (73.4294, 2.9952) centre (73.3171, 2.8829) ccw
  line L129 (74.2467, 2.8829) -> (73.3171, 2.8829)
  line L130 (73.3171, 2.8829) -> (72.39, 3.81)
  arc A261 (76.3123, 11.3177) -> (76.0877, 11.5423) centre (76.2, 11.43) ccw
  arc A262 (58.5787, 43.18) -> (58.2613, 43.18) centre (58.42, 43.18) ccw
  arc A263 (22.7477, 24.2423) -> (22.9723, 24.0177) centre (22.86, 24.13) ccw
  line L131 (22.86, 24.13) -> (24.13, 25.4)
  arc A264 (74.3311, 16.9017) -> (74.1065, 16.6771) centre (74.2188, 16.7894) ccw
  line L132 (74.93, 10.16) -> (76.2, 11.43)
  line L133 (63.5, 35.56) -> (58.42, 40.64)
  arc A265 (50.6413, 17.78) -> (50.9588, 17.78) centre (50.8001, 17.78) ccw
  arc A266 (76.0877, 14.6959) -> (76.3123, 14.9205) centre (76.2, 14.8082) ccw
  line L134 (13.97, 33.909) -> (15.24, 32.639)
  line L135 (63.5, 31.75) -> (63.5, 35.56)
  arc A267 (73.66, 10.3187) -> (73.66, 10.0013) centre (73.66, 10.16) ccw
  arc A268 (73.7723, 10.0477) -> (73.5477, 10.2723) centre (73.66, 10.16) ccw
  arc A269 (76.3588, 14.8082) -> (76.0413, 14.8082) centre (76.2001, 14.8082) ccw
  arc A270 (58.5323, 40.7523) -> (58.3077, 40.5277) centre (58.42, 40.64) ccw
  line L136 (15.24, 26.67) -> (16.002, 25.908)
  arc A271 (26.67, 25.2413) -> (26.67, 25.5588) centre (26.67, 25.4001) ccw
  arc A272 (58.2613, 40.64) -> (58.5787, 40.64) centre (58.42, 40.64) ccw
  arc A273 (24.13, 25.5588) -> (24.13, 25.2413) centre (24.13, 25.4001) ccw
  arc A274 (23.0188, 24.13) -> (22.7012, 24.13) centre (22.86, 24.13) ccw
  arc A275 (40.4813, 33.02) -> (40.7987, 33.02) centre (40.64, 33.02) ccw
  line L137 (40.64, 38.1) -> (40.64, 33.02)
  line L138 (24.13, 25.4) -> (26.67, 25.4)
  line L139 (15.24, 32.639) -> (15.24, 26.67)
  arc A276 (15.1277, 32.5267) -> (15.3523, 32.7513) centre (15.24, 32.639) ccw
  arc A277 (15.0813, 26.67) -> (15.3987, 26.67) centre (15.24, 26.67) ccw
  arc A278 (24.2423, 25.2877) -> (24.0177, 25.5123) centre (24.13, 25.4) ccw
  line L140 (58.42, 40.64) -> (58.42, 43.18)
  arc A279 (14.0823, 34.0213) -> (13.8577, 33.7967) centre (13.97, 33.909) ccw
  arc A280 (22.7012, 16.51) -> (23.0188, 16.51) centre (22.86, 16.51) ccw
  arc A281 (15.3987, 32.639) -> (15.0813, 32.639) centre (15.24, 32.639) ccw
sketch "Vias" plane through (0, 0, 0) normal (0, 0, 1) x (1, 0, 0)
  arc A0 (16.002, 25.6939) -> (16.002, 26.1221) centre (16.002, 25.908) ccw
  arc A1 (16.002, 26.1221) -> (16.002, 25.6939) centre (16.002, 25.908) ccw
  arc A2 (16.002, 25.6939) -> (16.002, 26.1221) centre (16.002, 25.908) ccw
  arc A3 (45.72, 14.1841) -> (45.72, 13.7559) centre (45.72, 13.97) ccw
  arc A4 (45.72, 13.7559) -> (45.72, 14.1841) centre (45.72, 13.97) ccw
  arc A5 (45.72, 14.1841) -> (45.72, 13.7559) centre (45.72, 13.97) ccw
  arc A6 (45.72, 13.7559) -> (45.72, 14.1841) centre (45.72, 13.97) ccw
  arc A7 (71.12, 39.1559) -> (71.12, 39.5841) centre (71.12, 39.37) ccw
  arc A8 (71.12, 39.1559) -> (71.12, 39.5841) centre (71.12, 39.37) ccw
  arc A9 (16.002, 26.1221) -> (16.002, 25.6939) centre (16.002, 25.908) ccw
  arc A10 (67.31, 16.2959) -> (67.31, 16.7241) centre (67.31, 16.51) ccw
  arc A11 (41.91, 25.1859) -> (41.91, 25.6141) centre (41.91, 25.4) ccw
  arc A12 (24.765, 28.9959) -> (24.765, 29.4241) centre (24.765, 29.21) ccw
  arc A13 (55.88, 34.5041) -> (55.88, 34.0759) centre (55.88, 34.29) ccw
  arc A14 (67.31, 10.3741) -> (67.31, 9.9459) centre (67.31, 10.16) ccw
  arc A15 (67.31, 9.9459) -> (67.31, 10.3741) centre (67.31, 10.16) ccw
  arc A16 (71.12, 37.0441) -> (71.12, 36.6159) centre (71.12, 36.83) ccw
  arc A17 (40.64, 30.2659) -> (40.64, 30.6941) centre (40.64, 30.48) ccw
  arc A18 (53.34, 44.2359) -> (53.34, 44.6641) centre (53.34, 44.45) ccw
  arc A19 (53.34, 44.2359) -> (53.34, 44.6641) centre (53.34, 44.45) ccw
  arc A20 (71.12, 36.6159) -> (71.12, 37.0441) centre (71.12, 36.83) ccw
  arc A21 (24.765, 45.5059) -> (24.765, 45.9341) centre (24.765, 45.72) ccw
  arc A22 (24.765, 45.9341) -> (24.765, 45.5059) centre (24.765, 45.72) ccw
  arc A23 (71.12, 39.5841) -> (71.12, 39.1559) centre (71.12, 39.37) ccw
  arc A24 (55.88, 34.0759) -> (55.88, 34.5041) centre (55.88, 34.29) ccw
  arc A25 (40.64, 30.2659) -> (40.64, 30.6941) centre (40.64, 30.48) ccw
  arc A26 (41.91, 25.6141) -> (41.91, 25.1859) centre (41.91, 25.4) ccw
  arc A27 (71.12, 36.6159) -> (71.12, 37.0441) centre (71.12, 36.83) ccw
  arc A28 (55.88, 34.5041) -> (55.88, 34.0759) centre (55.88, 34.29) ccw
  arc A29 (53.34, 44.6641) -> (53.34, 44.2359) centre (53.34, 44.45) ccw
  arc A30 (41.91, 25.6141) -> (41.91, 25.1859) centre (41.91, 25.4) ccw
  arc A31 (71.12, 39.5841) -> (71.12, 39.1559) centre (71.12, 39.37) ccw
  arc A32 (67.31, 16.7241) -> (67.31, 16.2959) centre (67.31, 16.51) ccw
  arc A33 (55.88, 34.0759) -> (55.88, 34.5041) centre (55.88, 34.29) ccw
  arc A34 (67.31, 9.9459) -> (67.31, 10.3741) centre (67.31, 10.16) ccw
  arc A35 (67.31, 16.7241) -> (67.31, 16.2959) centre (67.31, 16.51) ccw
  arc A36 (24.765, 29.4241) -> (24.765, 28.9959) centre (24.765, 29.21) ccw
  arc A37 (24.765, 45.5059) -> (24.765, 45.9341) centre (24.765, 45.72) ccw
  arc A38 (67.31, 16.2959) -> (67.31, 16.7241) centre (67.31, 16.51) ccw
  arc A39 (40.64, 30.6941) -> (40.64, 30.2659) centre (40.64, 30.48) ccw
  arc A40 (41.91, 25.1859) -> (41.91, 25.6141) centre (41.91, 25.4) ccw
  arc A41 (71.12, 37.0441) -> (71.12, 36.6159) centre (71.12, 36.83) ccw
  arc A42 (24.765, 29.4241) -> (24.765, 28.9959) centre (24.765, 29.21) ccw
  arc A43 (67.31, 10.3741) -> (67.31, 9.9459) centre (67.31, 10.16) ccw
  arc A44 (24.765, 45.9341) -> (24.765, 45.5059) centre (24.765, 45.72) ccw
  arc A45 (53.34, 44.6641) -> (53.34, 44.2359) centre (53.34, 44.45) ccw
  arc A46 (24.765, 28.9959) -> (24.765, 29.4241) centre (24.765, 29.21) ccw
  arc A47 (40.64, 30.6941) -> (40.64, 30.2659) centre (40.64, 30.48) ccw
extrude "Extrude3" add sketch "Outline" along normal blind 1.5 contours L0 L1 L2 L3 makes body 1
extrude "Extrude4" cut sketch "Vias" sketch "Through Holes" along normal through all of sketch 2 bodies 1
extrude "Extrude5" add sketch "Top Component Outlines" along normal blind 2 from surface at 1.5 separate body contours A0 A1 A2 A4 A6 A7 A8 A10 A11 L1 A13 L2 A14 A15 A16 L4 A17 A19 A22 A23 A24 A25 A26 L6 | A5 L0 L7 | L0 L3 A28 | A5 L3 A20 A28 L7 | L3 A20 L7 | A9 L5 L9 | L5 A29 L8 | A9 A27 A29 L8 L9 | A27 L8 L9 | L10 L11 L20 L25 L29 L30 | L10 L25 L30 L31 L33 | L20 L22 L25 L30 L34 | L12 A43 L23 A53 A55 | L12 L13 A49 A53 A55 A57 | A33 L13 L21 A49 A53 A57 | A43 L23 L28 A55 | A33 A43 L21 L24 A49 | A33 A43 L24 L28 | L19 A43 L23 L28 A55 | A33 L19 A43 L24 L28 | A214 L109 A215 L110 A216 A217 A218 L111 A219 A221 A224 A225 A230 A234 A235 L116 A237 A239 A240 A244 L119 L120 L121 A248 A249 A250 L122 A253 A254 A255 A256 A258 L124 L125 L126 L129 L131 A276 L137 A287 A289 A290 | A215 A216 L120 L126 | A249 L125 L126 A289 | L119 A253 A258 L124 | L110 A234 L119 A254 | A260 A261 A263 A265 L130 A266 A267 A268 A269 L132 L133 A271 A273 L134 L135 A275 A277 A278 A279 A280 A281 A282 L138 L139 A286 A288 L141 L142 L145 A291 A292 L146 A293 A294 A295 L148 L149 A296 A297 A298 L150 A299 | L130 A268 L133 A295 | A263 L133 L135 A279 | A269 L146 A296 L150 | A271 L138 A292 L146 | A300 A302 A303 A305 L152 A307 A308 L154 A309 A311 L155 A313 A314 L156 A315 L158 A317 L160 A318 A319 A320 A321 A322 A324 A325 A326 A327 A328 A329 L162 L163 L164 L165 A330 A331 L167 L169 L170 A334 L171 A337 A338 | A318 A324 L164 L167 | A320 A325 L165 L170 | A309 L156 A326 L167 | A303 L152 A317 L170 | A323 L161 A333 A339 A340 L173 L174 A341 A342 A343 A344 A347 L176 A348 A349 L178 A351 A352 A354 L181 A355 L183 A359 L185 L186 A360 A361 A362 A364 L188 L189 A367 A368 L190 A369 A370 L191 A371 L194 A376 A377 A378 | L161 A339 L173 A368 | L173 L178 A360 A369 | A354 L183 L185 A362 | A347 L183 L191 A376 | A353 L180 A357 A363 L187 A366 L193 A374 A384 A386 A388 A390 A391 L200 L202 L203 A393 A394 A395 L204 A399 L206 A401 L208 A403 A404 A407 A409 A410 L210 A411 A412 A413 L213 L214 A417 L215 A418 A419 A420 A421 L216 | A395 L204 L213 A417 | L187 A391 A407 L213 | L202 L203 A399 A413 | L180 L202 A420 A421 | A380 L197 A382 A383 L198 A387 L199 L201 A396 A397 A400 A402 A405 A408 L212 A414 A422 A423 L218 A424 A428 L227 A434 A435 A436 A438 A442 A445 A446 A447 L233 L234 L235 L236 A452 L237 A453 L240 A454 A455 A456 L243 | L197 A414 L236 A453 | L197 A435 A438 L237 | L212 A422 A442 L240 | L199 L212 A428 A447 | L219 A425 A426 L221 L222 A429 L224 A431 A432 L226 A433 A437 A439 A440 L229 A441 A443 L230 L232 L242 A457 A459 A461 L245 A462 A463 A464 L246 A466 A467 A469 L247 A471 A472 L251 A476 L253 A478 A484 A485 A487 A488 | L224 A443 L230 A478 | A425 L229 L232 A488 | L224 L251 A484 A485 | L222 A431 L229 A471 | L244 A458 A460 L248 A473 A474 L252 A477 L254 A479 A480 L256 A482 L257 L258 A489 L259 A491 L260 L261 A494 A495 A496 A497 A498 A499 A501 L263 A504 A508 A510 A511 A512 L265 L269 A517 A518 A521 A522 L272 A526 A529 | A480 L258 A501 L272 | A458 L248 L258 A504 | L254 A482 L261 A495 | A479 L261 A499 L269 | A492 L262 A503 A507 L264 L268 A514 A516 L270 A519 A520 L271 A523 A524 A525 A527 A528 A530 A532 A533 A535 A537 A538 A541 A542 L277 A544 L279 L281 A550 L287 A554 A555 L289 A563 L292 A565 L293 L295 L296 A567 A568 | A503 L287 L295 A567 | L264 A523 A554 L295 | L262 A514 A538 L296 | A519 L293 L296 A568 | A531 A534 A543 L276 A546 A549 A551 L284 A552 L285 L286 A556 A557 A558 A559 L290 A561 A562 L291 A564 L294 L298 A569 A570 L300 A572 A573 A574 A575 A579 A580 A581 A582 A583 L302 A585 A593 L305 L311 L315 A616 L317 | L284 L285 A558 A572 | L284 A561 L298 A585 | A546 A549 L294 L300 | A543 L291 L300 A579 makes body 2 at (10.9643, 14.9013, 1.5) makes body 3 at (76.7927, 12.7847, 1.5) makes body 4 at (46.5243, 42.2487, 1.5) makes body 5 at (46.5243, 38.4387, 1.5) makes body 6 at (64.3043, 25.0613, 1.5) makes body 7 at (9.3811, 11.0786, 1.5) makes body 8 at (72.9513, 49.9462, 3.5) makes body 9 at (78.2743, 25.0613, 1.5) makes body 10 at (32.5543, 41.5713, 1.5) makes body 11 at (44.9157, 33.3587, 1.5) makes body 12 at (62.6957, 20.6587, 1.5) makes body 13 at (13.5467, 39.6663, 1.5)
extrude "Extrude6" add sketch "Top Component Outlines" along normal blind 5 from surface at 1.5 separate body contours A171 A173 A228 A242 A637 A638 | A220 A222 A232 A238 A635 A636 makes body 14 at (5.2377, 6.5817, 4.8333) makes body 15 at (14.3573, 6.5539, 4.8333)
fillet "Fillet1" radius 1.5 12 edges at (5.054, 6.5912, 6.5) (3.6983, 5.7369, 6.5) (3.6983, 4.3977, 6.5) (5.0362, 3.5437, 6.5) (6.4224, 4.37, 6.5) (6.4304, 5.7489, 6.5) (13.9567, 6.6039, 6.5) (12.601, 5.7496, 6.5) (12.601, 4.4104, 6.5) (13.9389, 3.5564, 6.5) (15.3251, 4.3827, 6.5) (15.3331, 5.7616, 6.5) on bodies 14 15
extrude "Extrude7" add sketch "Top Component Outlines" along normal blind 7 from surface at 1.5 separate body contours A591 A606 | A597 A619 | A605 A613 makes body 16
extrude "Extrude8" add sketch "Top Component Outlines" along normal blind 9.9 from surface at 1.5 separate body contours L52 A94 A95 A97 L53 L54 L55 L57 L58 L59 A102 L60 A104 A107 L61 L62 L63 L64 A118 A123 L65 L66 A125 L67 L68 L69 L70 L71 L72 L73 L74 L75 L76 A134 A135 A136 L77 A139 A140 L78 A142 L79 A145 L80 A148 L81 A150 A152 A154 L82 L83 L84 L85 A157 A158 A160 L86 A163 L87 L88 L89 A176 L90 L91 L93 L94 L95 L96 A196 L98 L100 A204 L101 L103 L104 L106 L107 A213 | L92 L97 L99 L105 makes body 17 at (9.098, 37.3533, 8.1) makes body 18 at (41.0753, 16.3103, 1.5)
extrude "Extrude9" add sketch "Top Component Outlines" along normal blind 12.8 from surface at 1.5 separate body contours A37 L18 A56 L37 | L26 A56 A62 L37 | A37 L18 A64 L36 | L26 A62 A64 L36 | A38 A41 makes body 19
extrude "Extrude10" add sketch "Top Component Outlines" along normal blind 4.75 from surface at 1.5 separate body contours A586 L309 A628 A630 A633 A634 makes body 20
extrude "Extrude11" add sketch "Bottom Component Outlines" against normal blind 2.6 separate body contours L8 A32 L18 A42 A43 L22 L23 L24 L25 A48 L26 A49 A50 A51 A54 L27 L28 L29 A55 L30 L31 L32 L33 L34 L35 L36 L37 L38 L39 L40 A73 A75 L41 A76 A81 L42 L43 A83 L44 L45 A86 L46 A91 L47 L48 L49 A93 A94 A96 L50 A97 A98 A100 L51 L52 L53 L54 L55 A106 A107 A108 L56 L57 L58 A114 L59 L60 L61 L62 L63 A120 A123 L64 A127 L65 L66 A129 A130 A132 A133 L67 A136 L68 L69 L70 A139 L71 L72 L73 L74 L75 A145 L76 A147 A148 A149 L77 L78 A150 L79 L80 A155 L81 L82 L83 L84 L85 A163 L86 L87 L88 L89 L90 L91 L92 L93 A176 L94 A178 L95 A181 A185 L96 A187 L97 A190 L98 A191 L99 L100 L101 A195 L102 L103 L104 L105 L106 A203 L107 A204 L108 L109 A217 A218 A219 L110 A220 L111 | L0 A2 A6 A8 A11 L1 L2 L3 L4 A14 L5 A18 L6 L7 A21 L9 L10 A26 L11 L12 L13 L14 L15 L16 L17 A39 L19 L20 L21 A40 A222 L112 A225 L113 L114 L115 L116 A230 L117 A231 A232 L118 L119 L120 L121 A239 L122 L123 A246 A247 L124 L125 L126 L127 A252 A253 A254 L128 L129 A261 L130 A263 L131 L132 A267 L133 A270 A271 A273 L134 A277 L135 L136 L137 L138 L139 A280 L140 L141 L142 L143 A283 A286 A288 A291 A292 L144 A294 A295 L145 L146 L147 A304 L148 A306 A309 L149 A310 L150 A311 L151 L152 L153 L154 L155 A316 L156 A319 L157 L158 L159 L160 L161 L162 L163 L164 L165 L166 L167 L168 L169 L170 A333 A336 L171 A338 L172 A342 A343 A344 L173 L174 L175 L176 A351 L177 A355 L178 A356 A357 L179 A361 A362 L180 L181 L182 A366 L183 makes body 21 at (32.581, 6.5552, 0) makes body 22 at (61.399, 49.7352, 0)
sketch "Minimal Projection" plane through (0, 0, 0) normal (0, 0, 1) x (1, 0, 0)
  line L0 (0, 56.3) -> (0, 0)
  line L1 (0, 0) -> (85, 0)
  line L2 (85, 0) -> (85, 56.3)
  line L3 (85, 56.3) -> (0, 56.3)
  circle A0 centre (80.645, 51.943) radius 1.5875
  circle A1 centre (4.318, 51.943) radius 1.5875

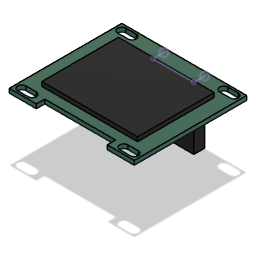
design "oled"
description: IIC OLED 0.96" 4Pin SSD1306
part number: GME12864-11
Autodesk Fusion 360 part; units mm, degrees